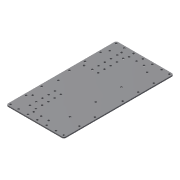
# Autodesk Inventor part: 足裏_アングル
Saved by Autodesk Inventor 2018.3 (Build 223284000, 284)
## iProperties
Category: 足先
Created: 2016-05-13
Part Number: 足裏_アングル
Material: GFRP
Document SubType Name: Modeling
Designer: hiroaki
Density: 1.75 g/cm^3
Appearance: 滑らか - 淡い灰色
Mass: 42.0096 g
Surface Area: 255.975 cm^2
Volume: 24.0055 cm^3
Author: hiroaki
Autodesk Inventor part; units mm, degrees
ref_plane "YZ Plane" through (0, 0, 0) normal (1, 0, 0) x (0, 1, 0)
ref_plane "XZ Plane" through (0, 0, 0) normal (0, 1, 0) x (-1, 0, 0)
ref_plane "XY Plane" through (0, 0, 0) normal (0, 0, 1) x (1, 0, 0)
sketch "スケッチ1" plane through (0, 0, 0) normal (0, 0, 1) x (1, 0, 0)
  circle A0 centre (-4.75, 50) radius 1.55
  circle A1 centre (4.75, 50) radius 1.55
  circle A2 centre (-4.75, -50) radius 1.55
  circle A3 centre (4.75, -50) radius 1.55
  line L0 (-4.75, -50) -> (4.75, -50) construction
  line L1 (4.75, -50) -> (4.75, 50) construction
  line L2 (4.75, 50) -> (-4.75, 50) construction
  line L3 (-4.75, 50) -> (-4.75, -50) construction
  line L4 (-4.75, -50) -> (4.75, 50) construction
  line L5 (4.75, -50) -> (-4.75, 50) construction
  circle A4 centre (4.75, 50) radius 2.75 construction
  circle A5 centre (-4.75, 40) radius 1.55
  circle A6 centre (4.75, 40) radius 1.55
  circle A7 centre (-4.75, -60) radius 1.55
  circle A8 centre (4.75, -60) radius 1.55
  circle A9 centre (-4.75, 30) radius 1.55
  circle A10 centre (4.75, 30) radius 1.55
  circle A11 centre (-4.75, -70) radius 1.55
  circle A12 centre (4.75, -70) radius 1.55
  circle A13 centre (-4.75, 20) radius 1.55
  circle A14 centre (4.75, 20) radius 1.55
  circle A15 centre (-4.75, -80) radius 1.55
  circle A16 centre (4.75, -80) radius 1.55
  circle A17 centre (-4.75, 10) radius 1.55
  circle A18 centre (4.75, 10) radius 1.55
  circle A19 centre (-4.75, -90) radius 1.55
  circle A20 centre (4.75, -90) radius 1.55
  line L6 (-25.25, 68.75) -> (67.25, 68.75)
  line L7 (67.25, 68.75) -> (67.25, -107.75)
  line L8 (67.25, -107.75) -> (-25.25, -107.75)
  line L9 (-25.25, -107.75) -> (-25.25, 68.75)
  circle A21 centre (63.75, 65.25) radius 1.55
  circle A22 centre (63.75, 40.25) radius 1.55
  circle A23 centre (63.75, 15.25) radius 1.55
  circle A24 centre (63.75, -9.75) radius 1.55
  line L10 (21, 59.3052) -> (21, 46.6028) construction
  circle A25 centre (63.75, -104.25) radius 1.55
  circle A26 centre (63.75, -79.25) radius 1.55
  circle A27 centre (63.75, -54.25) radius 1.55
  circle A28 centre (51.25, -104.25) radius 1.55
  circle A29 centre (36.25, -104.25) radius 1.55
  circle A30 centre (21.25, -104.25) radius 1.55
  circle A31 centre (6.25, -104.25) radius 1.55
  circle A32 centre (-8.75, -104.25) radius 1.55
  circle A33 centre (-21.75, -104.25) radius 1.55
  circle A34 centre (-21.75, -79.25) radius 1.55
  circle A35 centre (-21.75, -54.25) radius 1.55
  circle A36 centre (-21.75, 65.25) radius 1.55
  circle A37 centre (-21.75, 40.25) radius 1.55
  circle A38 centre (-21.75, 15.25) radius 1.55
  circle A39 centre (-21.75, -9.75) radius 1.55
  circle A40 centre (-4.75, 57) radius 1.55
  circle A41 centre (7.25, 57) radius 1.55
  circle A42 centre (19.25, 57) radius 1.55
  circle A43 centre (31.25, 57) radius 1.55
  circle A44 centre (43.25, -73.75) radius 1.55
  circle A45 centre (43.25, -32.5) radius 1.55
  circle A46 centre (43.25, 8.75) radius 1.55
  circle A47 centre (43.25, 50) radius 1.55
  circle A48 centre (7.25, -96) radius 1.55
  circle A49 centre (19.25, -96) radius 1.55
  circle A50 centre (31.25, -96) radius 1.55
  circle A51 centre (-16.75, -73.75) radius 1.55
  circle A52 centre (-16.75, -32.5) radius 1.55
  circle A53 centre (-16.75, 8.75) radius 1.55
  circle A54 centre (-16.75, 50) radius 1.55
  circle A55 centre (51.25, 65.25) radius 1.55
  circle A56 centre (36.25, 65.25) radius 1.55
  circle A57 centre (21.25, 65.25) radius 1.55
  circle A58 centre (6.25, 65.25) radius 1.55
  circle A59 centre (-8.75, 65.25) radius 1.55
  point P0 (0, 0)
  point P1 (0, 0)
  point P2 (0, 0)
  dimension "d0" = 3.1
  dimension "d1" = 9.5
  dimension "d2" = 100
  dimension "d41" = 5.5
  dimension "d47" = 10
  dimension "d54" = 92.5
  dimension "d55" = 176.5
  dimension "d56" = 3.1
  dimension "d59" = 25
  dimension "d79" = 20.5
  dimension "d80" = 57.75
  dimension "d83" = 3.5
  dimension "d84" = 3.5
  dimension "d99" = 3.1
  dimension "d100" = 3.5
  dimension "d101" = 3.5
  dimension "d104" = 25
  dimension "d110" = 3.1
  dimension "d111" = 12.5
  dimension "d114" = 15
  dimension "d119" = 3.1
  dimension "d120" = 3.5
  dimension "d123" = 25
  dimension "d128" = 3.1
  dimension "d129" = 3.5
  dimension "d130" = 3.5
  dimension "d133" = 25
  dimension "d138" = 3.5
  dimension "d139" = 3.5
  dimension "d140" = 3.1
  dimension "d141" = 20.5
  dimension "d142" = 11.75
  dimension "d145" = 12
  dimension "d150" = 3.1
  dimension "d151" = 24
  dimension "d152" = 34
  dimension "d155" = 41.25
  dimension "d160" = 3.1
  dimension "d161" = 11.75
  dimension "d162" = 32.5
  dimension "d165" = 12
  dimension "d170" = 3.1
  dimension "d171" = 34
  dimension "d172" = 8.5
  dimension "d175" = 41.25
  dimension "d180" = 3.1
  dimension "d181" = 3.5
  dimension "d182" = 12.5
  dimension "d185" = 15
  constraints: 60 centre point, 22 end point, 10 coincident, 9 vertical, 5 horizontal, 3 equal radius, 3 midpoint, 2 parallel, 96 other
  measures "d0" diameter of A1
  measures "d1" distance of L1.end L2.end
  measures "d2" distance of L0.end L1.end
  measures "d41" diameter of A4
  measures "d47" distance of A0.centre A5.centre
  measures "d54" distance between parallel lines of L9 L7
  measures "d55" distance between parallel lines of L6 L8
  measures "d56" diameter of A21
  measures "d59" distance of A21.centre A22.centre
  measures "d79" distance between parallel lines of L3 L9
  measures "d80" distance between parallel lines of L8 L0
  measures "d83" distance from line of L7 A21.centre
  measures "d84" distance from line of L6 A21.centre
  measures "d99" diameter of A25
  measures "d100" distance from line of A25.centre L7
  measures "d101" distance from line of A25.centre L8
  measures "d104" distance of A25.centre A26.centre
  measures "d110" diameter of A28
  measures "d111" distance of A25.centre A28.centre
  measures "d114" distance of A28.centre A29.centre
  measures "d119" diameter of A33
  measures "d120" distance from line of A33.centre L9
  measures "d123" distance of A33.centre A34.centre
  measures "d128" diameter of A36
  measures "d129" distance from line of A36.centre L6
  measures "d130" distance from line of A36.centre L9
  measures "d133" distance of A36.centre A37.centre
  measures "d138" distance from line of A33.centre L8
  measures "d139" distance from line of A28.centre L8
  measures "d140" diameter of A40
  measures "d141" distance from line of A40.centre L9
  measures "d142" distance from line of A40.centre L6
  measures "d145" distance of A40.centre A41.centre
  measures "d150" diameter of A44
  measures "d151" distance from line of A44.centre L7
  measures "d152" distance from line of A44.centre L8
  measures "d155" distance of A44.centre A45.centre
  measures "d160" diameter of A48
  measures "d161" distance from line of A48.centre L8
  measures "d162" distance from line of A48.centre L9
  measures "d165" distance of A48.centre A49.centre
  measures "d170" diameter of A51
  measures "d171" distance from line of A51.centre L8
  measures "d172" distance from line of A51.centre L9
  measures "d175" distance of A51.centre A52.centre
  measures "d180" diameter of A55
  measures "d181" distance from line of A55.centre L6
  measures "d182" distance of A21.centre A55.centre
  measures "d185" distance of A55.centre A56.centre
extrude "押し出し4" add sketch "スケッチ1" along normal blind 2
fillet "フィレット2" radius 3 4 edges at (-25.25, -107.75, 1) (67.25, -107.75, 1) (-25.25, 68.75, 1) (67.25, 68.75, 1)
equation "\"d1\" = d20"
equation "\"H_head\" = 28.5"
equation "\"H_leg\" = 199.5"
equation "\"足の面積\" = 12720.125"
equation "\"現在の面積\" = 11560"
equation "\"足_短辺\" = 68"
equation "\"円柱\" = 313.5"
equation "\"胴体中心から手先\" = 342"
equation "\"H_leg_1\" = 186.2"
equation "\"H_leg_MAX\" = 399"
equation "\"H_head_1\" = 26.6"
equation "\"H_head_MAX\" = 142.5"
equation "\"d20\" = 9.5"
